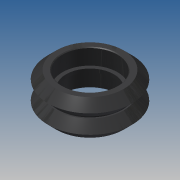
# Autodesk Inventor part: Delrin_Dual_V
Saved by Autodesk Inventor 2015 (Build 190159000, 159)
## iProperties
Created: 2015-01-09
Part Number: Delrin_Dual_V
Material: Generisch
Document SubType Name: Modeling
Designer: Marc
Density: 1 g/cm^3
Appearance: Dunkelgrau
Author: Marc
Autodesk Inventor part; units mm, degrees
ref_plane "YZ Plane" through (0, 0, 0) normal (1, 0, 0) x (0, 1, 0)
ref_plane "XZ Plane" through (0, 0, 0) normal (0, 1, 0) x (-1, 0, 0)
ref_plane "XY Plane" through (0, 0, 0) normal (0, 0, 1) x (1, 0, 0)
sketch "Skizze1" plane through (0, 0, 0) normal (0, 0, 1) x (1, 0, 0)
  line L0 (-17.073, 0) -> (17.073, 0) projected
  line L1 (0, -17.073) -> (0, 17.073) projected
  circle A0 centre (0, 0) radius 12.195
  dimension "d0" = 24.39
  constraints: 1 centre point, 1 coincident
  measures "d0" diameter of A0
extrude "Extrusion1" add sketch "Skizze1" along normal mid plane 10.23
sketch "Skizze2" plane through (0, 0, 5.115) normal (0, 0, 1) x (1, 0, 0)
  circle A0 centre (0, 0) radius 12.195 projected
  circle A1 centre (0, 0) radius 8
  dimension "d3" = 16
  constraints: 1 centre point, 1 coincident
  measures "d3" diameter of A1
extrude "Extrusion2" cut sketch "Skizze2" against normal blind 4.615 contours A1
chamfer "Fase1" distance 0.2 angle 45 1 edges at (-8, 0, 5.115)
mirror "Spiegeln1" about plane through (0, 0, 0) normal (0, 0, 1) of "Extrusion2"
chamfer "Fase2" distance 0.2 angle 45 1 edges at (-8, 0, -5.115)
sketch "Skizze3" plane through (0, 0, 0.5) normal (0, 0, 1) x (1, 0, 0)
  circle A0 centre (0, 0) radius 8 projected
  circle A1 centre (0, 0) radius 6.945
  dimension "d12" = 13.89
  constraints: 1 centre point, 1 coincident
  measures "d12" diameter of A1
extrude "Extrusion3" cut sketch "Skizze3" against normal blind 1 contours A1
sketch "Skizze4" plane through (0, 0, 0) normal (0, 1, 0) x (-1, 0, 0)
  line L0 (17.073, 0) -> (-17.073, 0) projected
  line L1 (0, -7.161) -> (0, 7.161) projected
  line L2 (-12.195, -5.115) -> (12.195, -5.115) projected
  line L3 (12.195, 5.115) -> (-12.195, 5.115) projected
  line L4 (-12.195, -5.115) -> (-12.195, 5.115) projected
  line L5 (-12.195, -5.115) -> (12.195, -5.115) projected
  line L6 (-9.7834, -5.115) -> (-12.195, -2.69)
  line L7 (-12.195, -2.69) -> (-9.77, -0.2784)
  line L8 (-9.77, -0.2784) -> (-9.375, -0.2784)
  line L9 (-9.375, -0.2784) -> (-9.375, 0.2784)
  line L10 (-9.375, 0.2784) -> (-9.7834, 0.2784)
  line L11 (-9.7834, 0.2784) -> (-12.195, 2.7034)
  line L12 (-12.195, 2.7034) -> (-9.77, 5.115)
  line L13 (12.195, 5.115) -> (-12.195, 5.115) projected
  point P0 (0, 0)
  dimension "d15" = 3.42
  dimension "d17" = 9.375
  dimension "d18" = 9.77
  constraints: 14 end point, 8 perpendicular, 4 point on line, 1 parallel
  measures "d15" distance of L6.start L6.end
  measures "d17" distance between parallel lines of L1 L9
  measures "d18" distance from line of L1 L7.end
revolve "Umdrehung1" cut sketch "Skizze4" angle 360 about axis through (0, 0, -10) along (0, 0, 1) contours L9 L8 L7 L4 L0 | L0 L4 L11 L10 L9 | L2 L4 L6 | L12 L4 L3
